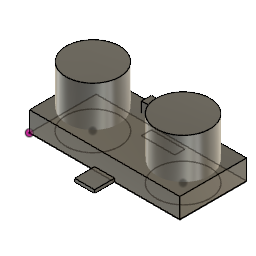
Capteur de distance v1 (Autodesk Fusion 360 design; units mm, degrees)
Autodesk Fusion 360 part; units mm, degrees
sketch "Sketch1" plane through (0, 0, 0) normal (0, 0, 1) x (1, 0, 0)
  line L0 (0, 0) -> (45, 0)
  line L1 (45, 0) -> (45, 20)
  line L2 (45, 20) -> (0, 20)
  line L3 (0, 20) -> (0, 0)
  line L4 (17.5, 19) -> (27.5, 19)
  line L5 (27.5, 19) -> (27.5, 16)
  line L6 (27.5, 16) -> (17.5, 16)
  line L7 (17.5, 16) -> (17.5, 19)
  circle A0 centre (9, 10) radius 8
  circle A1 centre (36, 10) radius 8
  dimension "d1" = 45
  dimension "d2" = 20
  dimension "d3" = 10
  dimension "d4" = 3
  dimension "d5" = 16
  dimension "d6" = 16
  dimension "d7" = 9
  dimension "d8" = 9
  dimension "d9" = 17.5
  dimension "d10" = 1
  dimension "d11" = 10
  dimension "d12" = 10
  measures "d5" diameter of A0
  measures "d6" diameter of A1
  measures "d9" distance of L3 L7
  measures "d10" distance of L2 L4
extrude "Extrude1" add sketch "Sketch1" along normal blind 6 contours L0 L1 L2 L3 | L4 L5 L6 L7 | A0 | A1 makes body 1
extrude "Extrude2" add sketch "Sketch1" along normal blind 18 separate body contours A0 makes body 2
extrude "Extrude3" add sketch "Sketch1" along normal blind 18 separate body contours A1 makes body 3
extrude "Extrude4" add sketch "Sketch1" along normal blind 9 separate body contours L4 L5 L6 L7 makes body 4
sketch "Sketch2" plane through (0, 0, 0) normal (0, -1, 0) x (1, 0, 0)
  line L0 (0, 0) -> (45, 0)
  line L1 (45, 0) -> (45, 6)
  line L2 (45, 6) -> (0, 6)
  line L3 (0, 6) -> (0, 0)
  line L4 (17.5, 0) -> (23.5, 0)
  line L5 (19.5, 0) -> (25.5, 0)
  line L6 (25.5, 0) -> (25.5, 1)
  line L7 (25.5, 1) -> (19.5, 1)
  line L8 (19.5, 1) -> (19.5, 0)
  dimension "d26" = 19.5
  measures "d26" distance of L3 L8
extrude "Extrude5" add sketch "Sketch2" along normal blind 6 contours L0 L4 L5 L6 L7 L8 bodies 1
